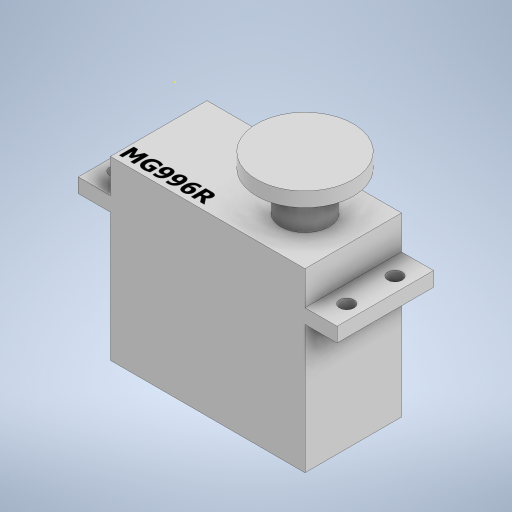
# Autodesk Inventor part: servo
Saved by Autodesk Inventor 2024.3 (Build 283343000, 343)
## iProperties
Created: 2024-10-22
Part Number: servo
Material: 一般
Document SubType Name: Modeling
Designer: 佐藤智貴
Density: 1 g/cm^3
Appearance: 既定
Project: MG996R
Author: 佐藤智貴
Title: MG996R
Autodesk Inventor part; units mm, degrees
ref_plane "YZ Plane" through (0, 0, 0) normal (1, 0, 0) x (0, 1, 0)
ref_plane "XZ Plane" through (0, 0, 0) normal (0, 1, 0) x (-1, 0, 0)
ref_plane "XY Plane" through (0, 0, 0) normal (0, 0, 1) x (1, 0, 0)
sketch "スケッチ1" plane through (0, 0, 0) normal (0, 0, 1) x (1, 0, 0)
  line L0 (0, 0) -> (53.6, 0)
  line L1 (53.6, 0) -> (53.6, 36.6)
  line L2 (53.6, 36.6) -> (0, 36.6)
  line L3 (0, 36.6) -> (0, 0)
  dimension "d2" = 36.6
  dimension "d3" = 53.6
  constraints: 8 end point, 2 parallel, 1 horizontal, 1 perpendicular
  measures "d2" distance between parallel lines of L0 L2
  measures "d3" distance between parallel lines of L3 L1
extrude "押し出し1" add sketch "スケッチ1" along normal blind 20
sketch "スケッチ2" plane through (0, 0, 20) normal (0, 0, 1) x (1, 0, 0)
  line L0 (53.6, 0) -> (53.6, 36.6) projected
  line L1 (0, 0) -> (53.6, 0) projected
  line L2 (53.6, 26.6) -> (46.95, 26.6)
  line L3 (46.95, 26.6) -> (46.95, 0)
  line L4 (46.95, 0) -> (53.6, 0)
  line L5 (53.6, 0) -> (53.6, 26.6)
  line L6 (0, 36.6) -> (0, 0) projected
  line L7 (0, 26.6) -> (6.65, 26.6)
  line L8 (6.65, 26.6) -> (6.65, 0)
  line L9 (6.65, 0) -> (0, 0)
  line L10 (0, 0) -> (0, 26.6)
  line L11 (53.6, 36.6) -> (0, 36.6) projected
  line L12 (0, 36.6) -> (6.65, 36.6)
  line L13 (6.65, 36.6) -> (6.65, 29.6)
  line L14 (6.65, 29.6) -> (0, 29.6)
  line L15 (0, 29.6) -> (0, 36.6)
  line L16 (53.6, 36.6) -> (46.95, 36.6)
  line L17 (46.95, 36.6) -> (46.95, 29.6)
  line L18 (46.95, 29.6) -> (53.6, 29.6)
  line L19 (53.6, 29.6) -> (53.6, 36.6)
  point P0 (0, 29.6)
  dimension "d4" = 6.65
  dimension "d5" = 6.65
  dimension "d6" = 26.6
  dimension "d7" = 26.6
  dimension "d8" = 3
  dimension "d9" = 6.65
  dimension "d10" = 6.65
  constraints: 32 end point, 8 parallel, 5 point on line, 4 horizontal, 4 perpendicular
  measures "d4" distance of L2.start L2.end
  measures "d5" distance of L7.start L7.end
  measures "d6" distance of L7.end L8.end
  measures "d7" distance of L2.end L3.end
  measures "d8" distance from line of L7.end L14
  measures "d9" distance between parallel lines of L6 L13
  measures "d10" distance between parallel lines of L0 L17
extrude "押し出し2" cut sketch "スケッチ2" against normal blind 20 contours L1 L3 L2 L0 | L18 L17 L11 L0 | L1 L6 L7 L8 | L13 L14 L6 L11
sketch "スケッチ3" plane through (6.65, 36.6, 0) normal (0, 1, 0) x (1, 0, 0)
  circle A0 centre (30.3, -10) radius 10
  line L0 (40.3, -20) -> (0, -20) projected
  line L1 (40.3, -20) -> (40.3, 0) projected
  circle A1 centre (30.3, -10) radius 5
  point P0 (-6.65, 0)
  dimension "d13" = 20
  dimension "d14" = 10
  dimension "d15" = 10
  dimension "d16" = 10
  constraints: 2 centre point, 1 coincident
  measures "d13" diameter of A0
  measures "d14" distance from line of L0 A0.centre
  measures "d15" distance from line of L1 A0.centre
  measures "d16" diameter of A1
extrude "押し出し3" add sketch "スケッチ3" along normal blind 8 contours A1
sketch "スケッチ4" plane through (36.95, 44.6, 10) normal (0, 1, 0) x (1, 0, 0)
  circle A0 centre (0, 0) radius 10
  point P0 (-36.95, 10)
  dimension "d19" = 20
  constraints: 1 centre point
  measures "d19" diameter of A0
extrude "押し出し4" add sketch "スケッチ4" along normal blind 3
sketch "スケッチ6" plane through (6.65, 36.6, 0) normal (0, 1, 0) x (1, 0, 0)
  line L0 (0.3829, -15.7977) -> (36.2463, -15.7977) construction
  line L1 (36.2463, -15.7977) -> (36.2463, -22.1498) construction
  line L2 (36.2463, -22.1498) -> (0.3829, -22.1498) construction
  line L3 (0.3829, -22.1498) -> (0.3829, -15.7977) construction
  point P0 (-6.65, 0)
  constraints: 2 other
sketch "スケッチ7" plane through (46.95, 29.6, 20) normal (0, 1, 0) x (1, 0, 0)
  line L0 (6.65, 20) -> (6.65, 0) projected
  line L1 (0, 20) -> (6.65, 20) projected
  line L2 (-46.95, 0) -> (-46.95, 20) projected
  line L3 (-46.95, 20) -> (-40.3, 20) projected
  line L4 (0, 0) -> (0, 20) projected
  point P0 (3.65, 15)
  point P1 (3.65, 5)
  point P2 (-43.95, 15)
  point P3 (-43.95, 5)
  dimension "d22" = 3
  dimension "d23" = 3
  dimension "d24" = 10
  dimension "d25" = 5
  dimension "d26" = 53.6
  dimension "d27" = 3
  dimension "d28" = 10
  dimension "d29" = 3
  dimension "d30" = 5
  dimension "d38" = 6.65
  measures "d22" distance from line of L0 point (3.65, 5)
  measures "d23" distance from line of L0 point (3.65, 15)
  measures "d24" distance of point (3.65, 5) point (3.65, 15)
  measures "d25" distance from line of L1 point (3.65, 15)
  measures "d26" distance between parallel lines of L0 L2
  measures "d27" distance from line of L2 point (-43.95, 15)
  measures "d28" distance of point (-43.95, 15) point (-43.95, 5)
  measures "d29" distance from line of L2 point (-43.95, 5)
  measures "d30" distance from line of L3 point (-43.95, 15)
  measures "d38" distance between parallel lines of L0 L4
hole "穴1" at (50.6, 29.6, 5) at (50.6, 29.6, 15) at (3, 29.6, 5) at (3, 29.6, 15) direction (0, -1, 0) diameter 3 end through all
equation "\"d5\" = d4"
equation "\"d7\" = d6"
equation "\"d23\" = d22"
equation "\"d27\" = d22"
equation "\"d28\" = d24"
equation "\"d29\" = d23"
equation "\"d30\" = d25"
